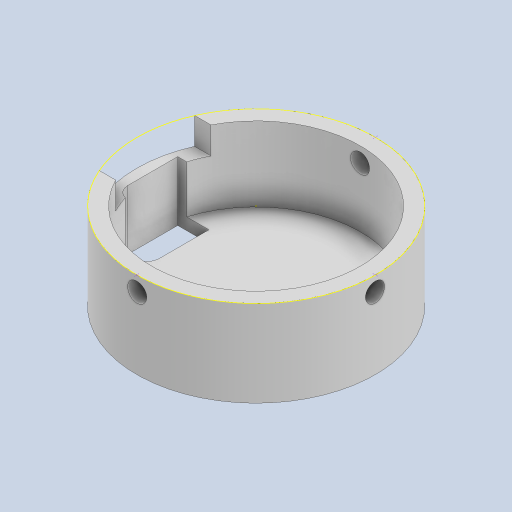
# Autodesk Inventor part: Payload Adapter
Saved by Autodesk Inventor 2024.2 (Build 282272000, 272)
## iProperties
Created: 2024-09-18
Part Number: Payload Adapter
Material: Generic
Document SubType Name: Modeling
Designer: Tom
Density: 1 g/cm^3
Appearance: Default
Author: Tom
Autodesk Inventor part; units mm, degrees
ref_plane "YZ Plane" through (0, 0, 0) normal (1, 0, 0) x (0, 1, 0)
sketch "Sketch1" plane through (0, 0, 0) normal (0, 1, 0) x (-1, 0, 0)
  circle A0 centre (0, 0) radius 20
  dimension "d0" = 40
  constraints: 1 centre point, 1 coincident
  measures "d0" diameter of A0
sketch "Sketch1 outline for Extrusion1" plane through (0, 0, 0) normal (0, 1, 0) x (-1, 0, 0)
  circle A0 centre (0, 0) radius 20
extrude "Extrusion1" add sketch "Sketch1 outline for Extrusion1" along normal blind 10
sketch "Sketch2" plane through (0, 10, 0) normal (0, 1, 0) x (1, 0, 0)
  circle A0 centre (0, 0) radius 17.5
  circle A1 centre (0, 0) radius 20
  line L0 (-18.330303, 8) -> (-15.564382, 8)
  line L1 (-18.330303, -8) -> (-15.564382, -8)
  circle A2 centre (0, 0) radius 20
  point P0 (-16.947343, 8)
  dimension "d3" = 35
  dimension "d4" = 8
  dimension "d5" = 8
  dimension "d6" = 40
  constraints: 4 end point, 4 point on circle, 2 centre point, 2 coincident, 1 horizontal, 1 midpoint, 1 parallel
  measures "d3" diameter of A0
  measures "d4" vertical distance of point (0, 0) point (-16.947, 8)
  measures "d5" distance from line of point (0, 0) L1
  measures "d6" diameter of A2
sketch "Sketch2 outline for Extrusion2" plane through (0, 10, 0) normal (0, 1, 0) x (1, 0, 0)
  line L0 (-15.564382, -8) -> (-18.330303, -8)
  arc A0 (-15.564382, 8) -> (-15.564382, -8) centre (0, 0) cw
  line L1 (-18.330303, 8) -> (-15.564382, 8)
  arc A1 (-18.330303, -8) -> (-18.330303, 8) centre (0, 0) ccw
extrude "Extrusion2" add sketch "Sketch2 outline for Extrusion2" along normal blind 4.5
sketch "Sketch3" plane through (0, 10, 0) normal (0, 1, 0) x (1, 0, 0)
  circle A0 centre (0, 0) radius 17.5
  constraints: 1 centre point, 1 coincident
sketch "Sketch3 outline for Extrusion3" plane through (0, 10, 0) normal (0, 1, 0) x (1, 0, 0)
  circle A0 centre (0, 0) radius 17.5
extrude "Extrusion3" cut sketch "Sketch3 outline for Extrusion3" against normal blind 8
sketch "Sketch4" plane through (0, 14.5, 0) normal (0, 1, 0) x (1, 0, 0)
  circle A0 centre (0, 0) radius 20 projected
  point P0 (0, -20.035453)
  point P1 (20, 0)
  point P2 (0, 20)
  constraints: 2 point on circle
ref_plane "Work Plane1" through (20, 14.5, 0) normal (1, 0, 0) x (0, 1, 0)
sketch "Sketch5" plane through (20, 14.5, 0) normal (1, 0, 0) x (0, 1, 0)
  circle A0 centre (-2.5, 0) radius 1.6
  line L0 (0, -20) -> (0, 20) projected
  point P0 (-14.5, 0)
  point P1 (0, 8)
  point P2 (0, -8)
  dimension "d11" = 3.2
  dimension "d12" = 2.5
  constraints: 1 centre point
  measures "d11" diameter of A0
  measures "d12" distance from line of L0 A0.centre
sketch "Sketch5 outline for Extrusion4" plane through (20, 14.5, 0) normal (1, 0, 0) x (0, 1, 0)
  circle A0 centre (-2.5, 0) radius 1.6
extrude "Extrusion4" cut sketch "Sketch5 outline for Extrusion4" against normal up to surface
ref_plane "Work Plane2" through (0, 14.5, -20) normal (0, 0, -1) x (-1, 0, 0)
sketch "Sketch6" plane through (0, 14.5, -20) normal (0, 0, -1) x (-1, 0, 0)
  circle A0 centre (0, -2.5) radius 1.6
  line L0 (18.330303, 0) -> (-20, 0)
  point P0 (0, -14.5)
  dimension "d15" = 3.2
  dimension "d16" = 2.5
  constraints: 1 centre point
  measures "d15" diameter of A0
  measures "d16" distance from line of L0 A0.centre
sketch "Sketch6 outline for Extrusion5" plane through (0, 14.5, -20) normal (0, 0, -1) x (-1, 0, 0)
  circle A0 centre (0, -2.5) radius 1.6
extrude "Extrusion5" cut sketch "Sketch6 outline for Extrusion5" against normal through all
sketch "Sketch7" plane through (0, 10, 0) normal (0, 1, 0) x (1, 0, 0)
  line L0 (-13, -3.3) -> (-13, 5.1)
  line L1 (-13, 5.1) -> (-18.25, 5.1)
  line L2 (-18.25, 5.1) -> (-18.25, -3.3)
  line L3 (-16.25, -5.3) -> (-15, -5.3)
  arc A0 (-15, -5.3) -> (-13, -3.3) centre (-15, -3.3) ccw
  arc A1 (-18.25, -3.3) -> (-16.25, -5.3) centre (-16.25, -3.3) ccw
  arc A2 (-18.330303, 8) -> (-18.330303, -8) centre (0, 0) ccw
  point P0 (-18.25, -5.3)
  dimension "d19" = 10.4
  dimension "d20" = 5.25
  dimension "d21" = 2
  dimension "d25" = 18.25
  dimension "d26" = 5.1
  constraints: 8 end point, 4 point on circle, 4 tangent, 2 centre point, 2 parallel, 2 point on line, 1 equal radius, 1 perpendicular
  measures "d19" distance of point (-18.25, -5.3) L1.end
  measures "d20" distance of L1.end L0.end
  measures "d21" radius of A0
  measures "d25" distance from line of L2 point (0, 0)
  measures "d26" distance from line of point (0, 0) L1
sketch "Sketch7 outline for Extrusion6" plane through (0, 10, 0) normal (0, 1, 0) x (1, 0, 0)
  line L0 (-13, -3.3) -> (-13, 5.1)
  arc A0 (-15, -5.3) -> (-13, -3.3) centre (-15, -3.3) ccw
  line L1 (-16.25, -5.3) -> (-15, -5.3)
  arc A1 (-18.25, -3.3) -> (-16.25, -5.3) centre (-16.25, -3.3) ccw
  line L2 (-18.25, 5.1) -> (-18.25, -3.3)
  line L3 (-13, 5.1) -> (-18.25, 5.1)
extrude "Extrusion6" cut sketch "Sketch7 outline for Extrusion6" against normal through all
body "Solid1"
